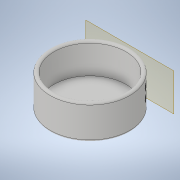
# Autodesk Inventor part: LargeFinderObjectiveCover-V02
Saved by Autodesk Inventor 2021.1 (Build 251245010, 245A)
## iProperties
Created: 2018-09-01
Part Number: LargeFinderObjectiveCover-V02
Material: Generic
Document SubType Name: Modeling
Designer: steele
Density: 1 g/cm^3
Appearance: Default
Author: steele
Autodesk Inventor part; units mm, degrees
ref_plane "YZ Plane" through (0, 0, 0) normal (1, 0, 0) x (0, 1, 0)
ref_plane "XZ Plane" through (0, 0, 0) normal (0, 1, 0) x (-1, 0, 0)
sketch "Sketch1" plane through (0, 0, 0) normal (0, 1, 0) x (-1, 0, 0)
  circle A0 centre (0, 0) radius 33.528
  dimension "d0" = 67.056
  constraints: 1 centre point, 1 coincident
  measures "d0" diameter of A0
extrude "Extrusion1" add sketch "Sketch1" along normal blind 3.175
sketch "Sketch2" plane through (0, 3.175, 0) normal (0, 1, 0) x (1, 0, 0)
  circle A0 centre (0, 0) radius 33.528
  circle A1 centre (0, 0) radius 30.353
  dimension "d4" = 60.706
  dimension "d5" = 67.056
  constraints: 2 centre point, 1 coincident
  measures "d4" diameter of A1
  measures "d5" diameter of A0
extrude "Extrusion3" add sketch "Sketch2" along normal blind 25.4
ref_plane "Work Plane1" through (0, 0, -33.528) normal (0, 0, 1) x (1, 0, 0)
sketch "Sketch5" plane through (0, 0, -33.528) normal (0, 0, 1) x (1, 0, 0)
  line L0 (-33.528, 0) -> (-33.528, 28.575) projected
  line L1 (33.528, 0) -> (33.528, 28.575) projected
  line L2 (33.528, 14.2875) -> (-33.528, 14.2875) construction
  line L3 (2.0888, 14.2875) -> (0.121, 14.2875)
  line L4 (0.121, 14.2875) -> (0.121, 13.7688)
  line L5 (0.121, 13.7688) -> (0.7674, 13.7688)
  line L6 (0.7674, 13.7688) -> (0.7674, 9.7262)
  line L7 (0.7674, 9.7262) -> (0.121, 9.7262)
  line L8 (0.121, 9.7262) -> (0.121, 9.2075)
  line L9 (0.121, 9.2075) -> (2.0888, 9.2075)
  line L10 (2.0888, 9.2075) -> (2.0888, 9.7262)
  line L11 (2.0888, 9.7262) -> (1.4425, 9.7262)
  line L12 (1.4425, 9.7262) -> (1.4425, 13.7688)
  line L13 (1.4425, 13.7688) -> (2.0888, 13.7688)
  line L14 (2.0888, 13.7688) -> (2.0888, 14.2875)
  spline S0 degree 2 poles (6.93, 11.7516) (6.93, 12.4473) (6.3661, 13.5671) (5.8926, 13.8799) knots 0 0 0 1 2 2 2
  spline S1 degree 2 poles (5.8926, 13.8799) (5.5057, 14.1228) (4.7111, 14.2875) (4.0936, 14.2875) knots 0 0 0 1 2 2 2
  line L15 (4.0936, 14.2875) -> (2.9245, 14.2875)
  line L16 (2.9245, 14.2875) -> (2.9245, 9.2075)
  line L17 (2.9245, 9.2075) -> (4.0813, 9.2075)
  spline S2 degree 2 poles (4.0813, 9.2075) (4.7976, 9.2075) (5.6127, 9.4216) (5.9009, 9.6109) knots 0 0 0 1 2 2 2
  spline S3 degree 2 poles (5.9009, 9.6109) (6.3908, 9.9362) (6.93, 11.0106) (6.93, 11.7516) knots 0 0 0 1 2 2 2
  spline S4 degree 2 poles (6.2261, 11.7434) (6.2261, 11.1588) (5.8391, 10.3314) (5.4563, 10.0967) knots 0 0 0 1 2 2 2
  spline S5 degree 2 poles (5.4563, 10.0967) (5.1846, 9.9362) (4.5712, 9.7921) (4.1142, 9.7921) knots 0 0 0 1 2 2 2
  line L18 (4.1142, 9.7921) -> (3.5996, 9.7921)
  line L19 (3.5996, 9.7921) -> (3.5996, 13.7029)
  line L20 (3.5996, 13.7029) -> (4.1142, 13.7029)
  spline S6 degree 2 poles (4.1142, 13.7029) (4.5629, 13.7029) (5.2422, 13.5588) (5.518, 13.3654) knots 0 0 0 1 2 2 2
  spline S7 degree 2 poles (5.518, 13.3654) (5.8721, 13.1266) (6.2261, 12.3362) (6.2261, 11.7434) knots 0 0 0 1 2 2 2
  line L21 (13.1545, 14.2875) -> (12.3394, 14.2875)
  line L22 (12.3394, 14.2875) -> (12.3394, 13.316)
  line L23 (12.3394, 13.316) -> (13.1545, 13.316)
  line L24 (13.1545, 13.316) -> (13.1545, 14.2875)
  line L25 (13.1545, 11.447) -> (12.3394, 11.447)
  line L26 (12.3394, 11.447) -> (12.3394, 10.4754)
  line L27 (12.3394, 10.4754) -> (13.1545, 10.4754)
  line L28 (13.1545, 10.4754) -> (13.1545, 11.447)
  line L29 (19.6671, 14.2875) -> (16.5343, 14.2875)
  line L30 (16.5343, 14.2875) -> (16.5343, 13.5671)
  spline S8 degree 2 poles (16.5343, 13.5671) (16.8719, 13.2501) (17.4729, 12.6614) (17.7611, 12.3444) knots 0 0 0 1 2 2 2
  spline S9 degree 2 poles (17.7611, 12.3444) (18.3415, 11.7063) (18.7655, 10.9406) (18.7655, 10.5331) knots 0 0 0 1 2 2 2
  spline S10 degree 2 poles (18.7655, 10.5331) (18.7655, 10.319) (18.6338, 9.9979) (18.5144, 9.895) knots 0 0 0 1 2 2 2
  spline S11 degree 2 poles (18.5144, 9.895) (18.395, 9.7921) (18.0822, 9.6892) (17.8928, 9.6892) knots 0 0 0 1 2 2 2
  spline S12 degree 2 poles (17.8928, 9.6892) (17.7117, 9.6892) (17.3412, 9.7797) (17.1724, 9.8497) knots 0 0 0 1 2 2 2
  spline S13 degree 2 poles (17.1724, 9.8497) (17.0283, 9.9073) (16.7607, 10.072) (16.6784, 10.1296) knots 0 0 0 1 2 2 2
  line L31 (16.6784, 10.1296) -> (16.6413, 10.1296)
  line L32 (16.6413, 10.1296) -> (16.6413, 9.4051)
  spline S14 degree 2 poles (16.6413, 9.4051) (16.8513, 9.3022) (17.6046, 9.1005) (17.9422, 9.1005) knots 0 0 0 1 2 2 2
  spline S15 degree 2 poles (17.9422, 9.1005) (18.6544, 9.1005) (19.4571, 9.8538) (19.4571, 10.496) knots 0 0 0 1 2 2 2
  spline S16 degree 2 poles (19.4571, 10.496) (19.4571, 10.7965) (19.3172, 11.2988) (19.1937, 11.5128) knots 0 0 0 1 2 2 2
  spline S17 degree 2 poles (19.1937, 11.5128) (19.0702, 11.7351) (18.712, 12.1715) (18.5144, 12.3815) knots 0 0 0 1 2 2 2
  spline S18 degree 2 poles (18.5144, 12.3815) (18.1933, 12.7314) (17.407, 13.4806) (17.1724, 13.6988) knots 0 0 0 1 2 2 2
  line L33 (17.1724, 13.6988) -> (19.6671, 13.6988)
  line L34 (19.6671, 13.6988) -> (19.6671, 14.2875)
  line L35 (21.4373, 14.2875) -> (20.6222, 14.2875)
  line L36 (20.6222, 14.2875) -> (20.6222, 13.316)
  line L37 (20.6222, 13.316) -> (21.4373, 13.316)
  line L38 (21.4373, 13.316) -> (21.4373, 14.2875)
  spline S19 degree 2 poles (23.8332, 9.6892) (23.6479, 9.6892) (23.2815, 9.7797) (23.1045, 9.8497) knots 0 0 0 1 2 2 2
  spline S20 degree 2 poles (23.1045, 9.8497) (22.9399, 9.9197) (22.697, 10.0679) (22.6023, 10.1338) knots 0 0 0 1 2 2 2
  line L39 (22.6023, 10.1338) -> (22.5611, 10.1338)
  line L40 (22.5611, 10.1338) -> (22.5611, 9.4133)
  spline S21 degree 2 poles (22.5611, 9.4133) (22.7834, 9.294) (23.545, 9.1005) (23.8867, 9.1005) knots 0 0 0 1 2 2 2
  spline S22 degree 2 poles (23.8867, 9.1005) (24.2325, 9.1005) (24.7471, 9.2404) (24.957, 9.3886) knots 0 0 0 1 2 2 2
  spline S23 degree 2 poles (24.957, 9.3886) (25.1793, 9.5492) (25.4099, 10.0144) (25.4099, 10.3272) knots 0 0 0 1 2 2 2
  spline S24 degree 2 poles (25.4099, 10.3272) (25.4099, 10.7471) (24.8582, 11.3811) (24.4713, 11.4634) knots 0 0 0 1 2 2 2
  line L41 (24.4713, 11.4634) -> (24.4713, 11.5128)
  spline S25 degree 2 poles (24.4713, 11.5128) (24.6318, 11.5458) (24.9982, 11.694) (25.1546, 11.8422) knots 0 0 0 1 2 2 2
  spline S26 degree 2 poles (25.1546, 11.8422) (25.3111, 11.9863) (25.5087, 12.4473) (25.5087, 12.7808) knots 0 0 0 1 2 2 2
  spline S27 degree 2 poles (25.5087, 12.7808) (25.5087, 13.1225) (25.274, 13.7029) (25.06, 13.9252) knots 0 0 0 1 2 2 2
  spline S28 degree 2 poles (25.06, 13.9252) (24.8377, 14.1558) (24.2078, 14.3945) (23.8085, 14.3945) knots 0 0 0 1 2 2 2
  spline S29 degree 2 poles (23.8085, 14.3945) (23.4256, 14.3945) (22.6764, 14.2093) (22.4212, 14.0817) knots 0 0 0 1 2 2 2
  line L42 (22.4212, 14.0817) -> (22.4212, 13.3612)
  line L43 (22.4212, 13.3612) -> (22.4706, 13.3612)
  spline S30 degree 2 poles (22.4706, 13.3612) (22.6846, 13.5177) (23.4092, 13.8058) (23.7673, 13.8058) knots 0 0 0 1 2 2 2
  spline S31 degree 2 poles (23.7673, 13.8058) (23.9773, 13.8058) (24.3972, 13.6741) (24.5371, 13.5218) knots 0 0 0 1 2 2 2
  spline S32 degree 2 poles (24.5371, 13.5218) (24.673, 13.3695) (24.8171, 13.0072) (24.8171, 12.7314) knots 0 0 0 1 2 2 2
  spline S33 degree 2 poles (24.8171, 12.7314) (24.8171, 12.4556) (24.6565, 12.0974) (24.5124, 11.9945) knots 0 0 0 1 2 2 2
  spline S34 degree 2 poles (24.5124, 11.9945) (24.3684, 11.8916) (23.9773, 11.8134) (23.7467, 11.8134) knots 0 0 0 1 2 2 2
  line L44 (23.7467, 11.8134) -> (23.4586, 11.8134)
  line L45 (23.4586, 11.8134) -> (23.4586, 11.2494)
  line L46 (23.4586, 11.2494) -> (23.685, 11.2494)
  spline S35 degree 2 poles (23.685, 11.2494) (24.1419, 11.2494) (24.7183, 10.813) (24.7183, 10.3972) knots 0 0 0 1 2 2 2
  spline S36 degree 2 poles (24.7183, 10.3972) (24.7183, 10.2037) (24.5701, 9.9279) (24.4507, 9.8456) knots 0 0 0 1 2 2 2
  spline S37 degree 2 poles (24.4507, 9.8456) (24.3231, 9.7591) (24.0102, 9.6892) (23.8332, 9.6892) knots 0 0 0 1 2 2 2
  spline S38 degree 2 poles (26.1344, 10.8583) (26.1344, 10.4672) (26.3897, 9.8168) (26.612, 9.5821) knots 0 0 0 1 2 2 2
  spline S39 degree 2 poles (26.612, 9.5821) (26.8219, 9.3557) (27.4353, 9.1046) (27.7482, 9.1046) knots 0 0 0 1 2 2 2
  spline S40 degree 2 poles (27.7482, 9.1046) (28.0981, 9.1046) (28.6662, 9.3392) (28.8761, 9.5615) knots 0 0 0 1 2 2 2
  spline S41 degree 2 poles (28.8761, 9.5615) (29.1396, 9.8415) (29.4278, 10.7471) (29.4278, 11.4429) knots 0 0 0 1 2 2 2
  spline S42 degree 2 poles (29.4278, 11.4429) (29.4278, 12.0727) (29.1437, 13.2007) (28.8679, 13.5753) knots 0 0 0 1 2 2 2
  spline S43 degree 2 poles (28.8679, 13.5753) (28.5756, 13.9705) (27.7523, 14.3863) (27.1512, 14.3863) knots 0 0 0 1 2 2 2
  spline S44 degree 2 poles (27.1512, 14.3863) (27.0154, 14.3863) (26.7066, 14.3575) (26.5749, 14.3163) knots 0 0 0 1 2 2 2
  line L47 (26.5749, 14.3163) -> (26.5749, 13.6618)
  line L48 (26.5749, 13.6618) -> (26.6078, 13.6618)
  spline S45 degree 2 poles (26.6078, 13.6618) (26.6943, 13.7112) (27.0566, 13.7976) (27.2418, 13.7976) knots 0 0 0 1 2 2 2
  spline S46 degree 2 poles (27.2418, 13.7976) (27.9087, 13.7976) (28.6703, 12.9166) (28.7238, 12.1015) knots 0 0 0 1 2 2 2
  spline S47 degree 2 poles (28.7238, 12.1015) (28.4521, 12.2868) (27.9581, 12.4556) (27.6658, 12.4556) knots 0 0 0 1 2 2 2
  spline S48 degree 2 poles (27.6658, 12.4556) (27.3859, 12.4556) (26.9207, 12.3321) (26.6861, 12.1551) knots 0 0 0 1 2 2 2
  spline S49 degree 2 poles (26.6861, 12.1551) (26.4144, 11.9451) (26.1344, 11.307) (26.1344, 10.8583) knots 0 0 0 1 2 2 2
  spline S50 degree 2 poles (28.7403, 11.2905) (28.7403, 10.776) (28.5509, 10.1255) (28.3821, 9.9485) knots 0 0 0 1 2 2 2
  spline S51 degree 2 poles (28.3821, 9.9485) (28.2339, 9.7838) (27.9252, 9.6603) (27.744, 9.6603) knots 0 0 0 1 2 2 2
  spline S52 degree 2 poles (27.744, 9.6603) (27.3241, 9.6603) (26.826, 10.2614) (26.826, 10.8295) knots 0 0 0 1 2 2 2
  spline S53 degree 2 poles (26.826, 10.8295) (26.826, 11.1506) (26.9907, 11.5664) (27.1718, 11.7146) knots 0 0 0 1 2 2 2
  spline S54 degree 2 poles (27.1718, 11.7146) (27.3036, 11.8216) (27.6288, 11.8916) (27.8181, 11.8916) knots 0 0 0 1 2 2 2
  spline S55 degree 2 poles (27.8181, 11.8916) (28.0363, 11.8916) (28.5386, 11.7393) (28.7279, 11.6116) knots 0 0 0 1 2 2 2
  spline S56 degree 2 poles (28.7279, 11.6116) (28.7321, 11.5622) (28.7403, 11.3935) (28.7403, 11.2905) knots 0 0 0 1 2 2 2
  spline S57 degree 2 poles (33.2481, 11.7475) (33.2481, 13.1142) (32.4535, 14.3945) (31.6261, 14.3945) knots 0 0 0 1 2 2 2
  spline S58 degree 2 poles (31.6261, 14.3945) (30.7863, 14.3945) (30, 13.0895) (30, 11.7516) knots 0 0 0 1 2 2 2
  spline S59 degree 2 poles (30, 11.7516) (30, 10.3766) (30.7945, 9.1046) (31.6261, 9.1046) knots 0 0 0 1 2 2 2
  spline S60 degree 2 poles (31.6261, 9.1046) (32.4618, 9.1046) (33.2481, 10.4219) (33.2481, 11.7475) knots 0 0 0 1 2 2 2
  spline S61 degree 2 poles (32.3753, 13.2954) (32.4741, 13.0443) (32.5565, 12.2703) (32.5565, 11.7475) knots 0 0 0 1 2 2 2
  spline S62 degree 2 poles (32.5565, 11.7475) (32.5565, 11.2247) (32.4741, 10.4549) (32.3712, 10.1955) knots 0 0 0 1 2 2 2
  spline S63 degree 2 poles (32.3712, 10.1955) (32.2683, 9.9362) (31.9101, 9.6686) (31.6261, 9.6686) knots 0 0 0 1 2 2 2
  spline S64 degree 2 poles (31.6261, 9.6686) (31.342, 9.6686) (30.9756, 9.9362) (30.8686, 10.2037) knots 0 0 0 1 2 2 2
  spline S65 degree 2 poles (30.8686, 10.2037) (30.7657, 10.4631) (30.6916, 11.2535) (30.6916, 11.7516) knots 0 0 0 1 2 2 2
  spline S66 degree 2 poles (30.6916, 11.7516) (30.6916, 12.2868) (30.7575, 13.0031) (30.8645, 13.283) knots 0 0 0 1 2 2 2
  spline S67 degree 2 poles (30.8645, 13.283) (30.9633, 13.5465) (31.3297, 13.8305) (31.6261, 13.8305) knots 0 0 0 1 2 2 2
  spline S68 degree 2 poles (31.6261, 13.8305) (31.906, 13.8305) (32.2724, 13.563) (32.3753, 13.2954) knots 0 0 0 1 2 2 2
  spline S69 degree 2 poles (3.7561, 18.1769) (4.0442, 18.5144) (4.3653, 19.5024) (4.3653, 20.1364) knots 0 0 0 1 2 2 2
  spline S70 degree 2 poles (4.3653, 20.1364) (4.3653, 20.7539) (4.0525, 21.7543) (3.7561, 22.0918) knots 0 0 0 1 2 2 2
  spline S71 degree 2 poles (3.7561, 22.0918) (3.4432, 22.4459) (2.6157, 22.7834) (2.1176, 22.7834) knots 0 0 0 1 2 2 2
  spline S72 degree 2 poles (2.1176, 22.7834) (1.603, 22.7834) (0.7797, 22.4335) (0.4792, 22.0918) knots 0 0 0 1 2 2 2
  spline S73 degree 2 poles (0.4792, 22.0918) (0.1869, 21.7543) (-0.126, 20.7621) (-0.126, 20.1364) knots 0 0 0 1 2 2 2
  spline S74 degree 2 poles (-0.126, 20.1364) (-0.126, 19.4983) (0.191, 18.5268) (0.4833, 18.1769) knots 0 0 0 1 2 2 2
  spline S75 degree 2 poles (0.4833, 18.1769) (0.7797, 17.8393) (1.6072, 17.4894) (2.1176, 17.4894) knots 0 0 0 1 2 2 2
  spline S76 degree 2 poles (2.1176, 17.4894) (2.6363, 17.4894) (3.4679, 17.8516) (3.7561, 18.1769) knots 0 0 0 1 2 2 2
  spline S77 degree 2 poles (3.6614, 20.1364) (3.6614, 19.6342) (3.4432, 18.8561) (3.2456, 18.6009) knots 0 0 0 1 2 2 2
  spline S78 degree 2 poles (3.2456, 18.6009) (3.0439, 18.3374) (2.4758, 18.0739) (2.1217, 18.0739) knots 0 0 0 1 2 2 2
  spline S79 degree 2 poles (2.1217, 18.0739) (1.7554, 18.0739) (1.2037, 18.3292) (0.9938, 18.6009) knots 0 0 0 1 2 2 2
  spline S80 degree 2 poles (0.9938, 18.6009) (0.7921, 18.8602) (0.578, 19.6424) (0.578, 20.1364) knots 0 0 0 1 2 2 2
  spline S81 degree 2 poles (0.578, 20.1364) (0.578, 21.1368) (1.4178, 22.1989) (2.1217, 22.1989) knots 0 0 0 1 2 2 2
  spline S82 degree 2 poles (2.1217, 22.1989) (2.8257, 22.1989) (3.6614, 21.1368) (3.6614, 20.1364) knots 0 0 0 1 2 2 2
  spline S83 degree 2 poles (9.1119, 20.1405) (9.1119, 20.8362) (8.5479, 21.956) (8.0745, 22.2689) knots 0 0 0 1 2 2 2
  spline S84 degree 2 poles (8.0745, 22.2689) (7.6875, 22.5117) (6.893, 22.6764) (6.2755, 22.6764) knots 0 0 0 1 2 2 2
  line L49 (6.2755, 22.6764) -> (5.1063, 22.6764)
  line L50 (5.1063, 22.6764) -> (5.1063, 17.5964)
  line L51 (5.1063, 17.5964) -> (6.2631, 17.5964)
  spline S85 degree 2 poles (6.2631, 17.5964) (6.9794, 17.5964) (7.7945, 17.8105) (8.0827, 17.9998) knots 0 0 0 1 2 2 2
  spline S86 degree 2 poles (8.0827, 17.9998) (8.5726, 18.3251) (9.1119, 19.3995) (9.1119, 20.1405) knots 0 0 0 1 2 2 2
  spline S87 degree 2 poles (8.4079, 20.1323) (8.4079, 19.5477) (8.021, 18.7203) (7.6381, 18.4856) knots 0 0 0 1 2 2 2
  spline S88 degree 2 poles (7.6381, 18.4856) (7.3664, 18.3251) (6.753, 18.181) (6.2961, 18.181) knots 0 0 0 1 2 2 2
  line L52 (6.2961, 18.181) -> (5.7815, 18.181)
  line L53 (5.7815, 18.181) -> (5.7815, 22.0918)
  line L54 (5.7815, 22.0918) -> (6.2961, 22.0918)
  spline S89 degree 2 poles (6.2961, 22.0918) (6.7448, 22.0918) (7.424, 21.9478) (7.6999, 21.7543) knots 0 0 0 1 2 2 2
  spline S90 degree 2 poles (7.6999, 21.7543) (8.0539, 21.5155) (8.4079, 20.7251) (8.4079, 20.1323) knots 0 0 0 1 2 2 2
  line L55 (13.1545, 22.6764) -> (12.3394, 22.6764)
  line L56 (12.3394, 22.6764) -> (12.3394, 21.7049)
  line L57 (12.3394, 21.7049) -> (13.1545, 21.7049)
  line L58 (13.1545, 21.7049) -> (13.1545, 22.6764)
  line L59 (13.1545, 19.8359) -> (12.3394, 19.8359)
  line L60 (12.3394, 19.8359) -> (12.3394, 18.8643)
  line L61 (12.3394, 18.8643) -> (13.1545, 18.8643)
  line L62 (13.1545, 18.8643) -> (13.1545, 19.8359)
  line L63 (19.6671, 22.6764) -> (16.5343, 22.6764)
  line L64 (16.5343, 22.6764) -> (16.5343, 21.956)
  spline S91 degree 2 poles (16.5343, 21.956) (16.8719, 21.639) (17.4729, 21.0503) (17.7611, 20.7333) knots 0 0 0 1 2 2 2
  spline S92 degree 2 poles (17.7611, 20.7333) (18.3415, 20.0952) (18.7655, 19.3295) (18.7655, 18.922) knots 0 0 0 1 2 2 2
  spline S93 degree 2 poles (18.7655, 18.922) (18.7655, 18.7079) (18.6338, 18.3868) (18.5144, 18.2839) knots 0 0 0 1 2 2 2
  spline S94 degree 2 poles (18.5144, 18.2839) (18.395, 18.181) (18.0822, 18.0781) (17.8928, 18.0781) knots 0 0 0 1 2 2 2
  spline S95 degree 2 poles (17.8928, 18.0781) (17.7117, 18.0781) (17.3412, 18.1686) (17.1724, 18.2386) knots 0 0 0 1 2 2 2
  spline S96 degree 2 poles (17.1724, 18.2386) (17.0283, 18.2962) (16.7607, 18.4609) (16.6784, 18.5185) knots 0 0 0 1 2 2 2
  line L65 (16.6784, 18.5185) -> (16.6413, 18.5185)
  line L66 (16.6413, 18.5185) -> (16.6413, 17.794)
  spline S97 degree 2 poles (16.6413, 17.794) (16.8513, 17.6911) (17.6046, 17.4894) (17.9422, 17.4894) knots 0 0 0 1 2 2 2
  spline S98 degree 2 poles (17.9422, 17.4894) (18.6544, 17.4894) (19.4571, 18.2427) (19.4571, 18.8849) knots 0 0 0 1 2 2 2
  spline S99 degree 2 poles (19.4571, 18.8849) (19.4571, 19.1854) (19.3172, 19.6877) (19.1937, 19.9018) knots 0 0 0 1 2 2 2
  spline S100 degree 2 poles (19.1937, 19.9018) (19.0702, 20.1241) (18.712, 20.5604) (18.5144, 20.7704) knots 0 0 0 1 2 2 2
  spline S101 degree 2 poles (18.5144, 20.7704) (18.1933, 21.1203) (17.407, 21.8695) (17.1724, 22.0877) knots 0 0 0 1 2 2 2
  line L67 (17.1724, 22.0877) -> (19.6671, 22.0877)
  line L68 (19.6671, 22.0877) -> (19.6671, 22.6764)
  line L69 (21.4373, 22.6764) -> (20.6222, 22.6764)
  line L70 (20.6222, 22.6764) -> (20.6222, 21.7049)
  line L71 (20.6222, 21.7049) -> (21.4373, 21.7049)
  line L72 (21.4373, 21.7049) -> (21.4373, 22.6764)
  spline S102 degree 2 poles (25.6733, 21.0297) (25.6733, 21.4208) (25.414, 22.0836) (25.1958, 22.3059) knots 0 0 0 1 2 2 2
  spline S103 degree 2 poles (25.1958, 22.3059) (24.9694, 22.5406) (24.4013, 22.7834) (24.0596, 22.7834) knots 0 0 0 1 2 2 2
  spline S104 degree 2 poles (24.0596, 22.7834) (23.7179, 22.7834) (23.1539, 22.5529) (22.9399, 22.3224) knots 0 0 0 1 2 2 2
  spline S105 degree 2 poles (22.9399, 22.3224) (22.6764, 22.0466) (22.38, 21.1203) (22.38, 20.4452) knots 0 0 0 1 2 2 2
  spline S106 degree 2 poles (22.38, 20.4452) (22.38, 19.7824) (22.6517, 18.7161) (22.9357, 18.3209) knots 0 0 0 1 2 2 2
  spline S107 degree 2 poles (22.9357, 18.3209) (23.2116, 17.934) (24.0843, 17.5017) (24.6565, 17.5017) knots 0 0 0 1 2 2 2
  spline S108 degree 2 poles (24.6565, 17.5017) (24.8253, 17.5017) (25.1217, 17.5347) (25.2329, 17.5717) knots 0 0 0 1 2 2 2
  line L73 (25.2329, 17.5717) -> (25.2329, 18.2263)
  line L74 (25.2329, 18.2263) -> (25.204, 18.2263)
  spline S109 degree 2 poles (25.204, 18.2263) (25.1094, 18.1769) (24.7636, 18.0904) (24.566, 18.0904) knots 0 0 0 1 2 2 2
  spline S110 degree 2 poles (24.566, 18.0904) (23.932, 18.0904) (23.1539, 18.9467) (23.0798, 19.7865) knots 0 0 0 1 2 2 2
  spline S111 degree 2 poles (23.0798, 19.7865) (23.3227, 19.6177) (23.8332, 19.4325) (24.1378, 19.4325) knots 0 0 0 1 2 2 2
  spline S112 degree 2 poles (24.1378, 19.4325) (24.4342, 19.4325) (24.8788, 19.5518) (25.1217, 19.733) knots 0 0 0 1 2 2 2
  spline S113 degree 2 poles (25.1217, 19.733) (25.4016, 19.9429) (25.6733, 20.5934) (25.6733, 21.0297) knots 0 0 0 1 2 2 2
  spline S114 degree 2 poles (24.9817, 21.0585) (24.9817, 20.7457) (24.8171, 20.3217) (24.6359, 20.1735) knots 0 0 0 1 2 2 2
  spline S115 degree 2 poles (24.6359, 20.1735) (24.5001, 20.0664) (24.1625, 19.9964) (23.9855, 19.9964) knots 0 0 0 1 2 2 2
  spline S116 degree 2 poles (23.9855, 19.9964) (23.7467, 19.9964) (23.298, 20.1405) (23.0798, 20.2764) knots 0 0 0 1 2 2 2
  spline S117 degree 2 poles (23.0798, 20.2764) (23.0757, 20.3505) (23.0675, 20.4904) (23.0675, 20.5975) knots 0 0 0 1 2 2 2
  spline S118 degree 2 poles (23.0675, 20.5975) (23.0675, 21.1244) (23.2733, 21.7707) (23.4298, 21.9395) knots 0 0 0 1 2 2 2
  spline S119 degree 2 poles (23.4298, 21.9395) (23.5738, 22.1001) (23.8867, 22.2277) (24.0637, 22.2277) knots 0 0 0 1 2 2 2
  spline S120 degree 2 poles (24.0637, 22.2277) (24.4754, 22.2277) (24.9817, 21.6431) (24.9817, 21.0585) knots 0 0 0 1 2 2 2
  line L75 (29.543, 20.9309) -> (28.9379, 20.9309)
  line L76 (28.9379, 20.9309) -> (28.9379, 22.6764)
  line L77 (28.9379, 22.6764) -> (28.2833, 22.6764)
  line L78 (28.2833, 22.6764) -> (28.2833, 20.9309)
  line L79 (28.2833, 20.9309) -> (26.0397, 20.9309)
  line L80 (26.0397, 20.9309) -> (26.0397, 20.2146)
  line L81 (26.0397, 20.2146) -> (28.3121, 17.5964)
  line L82 (28.3121, 17.5964) -> (28.9379, 17.5964)
  line L83 (28.9379, 17.5964) -> (28.9379, 20.3834)
  line L84 (28.9379, 20.3834) -> (29.543, 20.3834)
  line L85 (29.543, 20.3834) -> (29.543, 20.9309)
  line L86 (28.2833, 20.3834) -> (28.2833, 18.3992)
  line L87 (28.2833, 18.3992) -> (26.5749, 20.3834)
  line L88 (26.5749, 20.3834) -> (28.2833, 20.3834)
  spline S121 degree 2 poles (33.2481, 20.1364) (33.2481, 21.5031) (32.4535, 22.7834) (31.6261, 22.7834) knots 0 0 0 1 2 2 2
  spline S122 degree 2 poles (31.6261, 22.7834) (30.7863, 22.7834) (30, 21.4784) (30, 20.1405) knots 0 0 0 1 2 2 2
  spline S123 degree 2 poles (30, 20.1405) (30, 18.7655) (30.7945, 17.4935) (31.6261, 17.4935) knots 0 0 0 1 2 2 2
  spline S124 degree 2 poles (31.6261, 17.4935) (32.4618, 17.4935) (33.2481, 18.8108) (33.2481, 20.1364) knots 0 0 0 1 2 2 2
  spline S125 degree 2 poles (32.3753, 21.6843) (32.4741, 21.4332) (32.5565, 20.6592) (32.5565, 20.1364) knots 0 0 0 1 2 2 2
  spline S126 degree 2 poles (32.5565, 20.1364) (32.5565, 19.6136) (32.4741, 18.8438) (32.3712, 18.5844) knots 0 0 0 1 2 2 2
  spline S127 degree 2 poles (32.3712, 18.5844) (32.2683, 18.3251) (31.9101, 18.0575) (31.6261, 18.0575) knots 0 0 0 1 2 2 2
  spline S128 degree 2 poles (31.6261, 18.0575) (31.342, 18.0575) (30.9757, 18.3251) (30.8686, 18.5926) knots 0 0 0 1 2 2 2
  spline S129 degree 2 poles (30.8686, 18.5926) (30.7657, 18.852) (30.6916, 19.6424) (30.6916, 20.1405) knots 0 0 0 1 2 2 2
  spline S130 degree 2 poles (30.6916, 20.1405) (30.6916, 20.6757) (30.7575, 21.392) (30.8645, 21.6719) knots 0 0 0 1 2 2 2
  spline S131 degree 2 poles (30.8645, 21.6719) (30.9633, 21.9354) (31.3297, 22.2195) (31.6261, 22.2195) knots 0 0 0 1 2 2 2
  spline S132 degree 2 poles (31.6261, 22.2195) (31.906, 22.2195) (32.2724, 21.9519) (32.3753, 21.6843) knots 0 0 0 1 2 2 2
  point P0 (0, 0)
  dimension "d9" = 25.4
  constraints: 2 end point, 2 midpoint, 1 horizontal
emboss "Emboss1" sketch "Sketch5" operation cut depth 1.27 direction (0, 0, -1) wrap yes faces at (-33.0938, 10.5833, -5.3783)
fillet "Fillet1" radius 1.5875 2 edges at (-33.528, 28.575, 0) (-30.353, 28.575, 0)
fillet "Fillet2" radius 1.5875 1 edges at (33.528, 0, 0)
equation "\"d0\" = lensCoverOD"
equation "\"d2\" = wallThickness"
equation "\"d4\" = lensCoverID"
equation "\"d5\" = lensCoverOD"
equation "\"d9\" = lensCoverLength"
equation "\"d11\" = textDepth"
equation "\"d13\" = filetRadius"
equation "\"d14\" = filetRadius"
equation "\"objectiveOD\" = 60.325"
equation "\"lensCoverLength\" = 25.4"
equation "\"wallThickness\" = 3.175"
equation "\"lensCoverOD\" = lensCoverID + 2 * wallThickness"
equation "\"clearance\" = 0.381"
equation "\"lensCoverID\" = objectiveOD + clearance"
equation "\"textDepth\" = 1.27"
equation "\"filetRadius\" = 1.5875"
body "Solid1"
